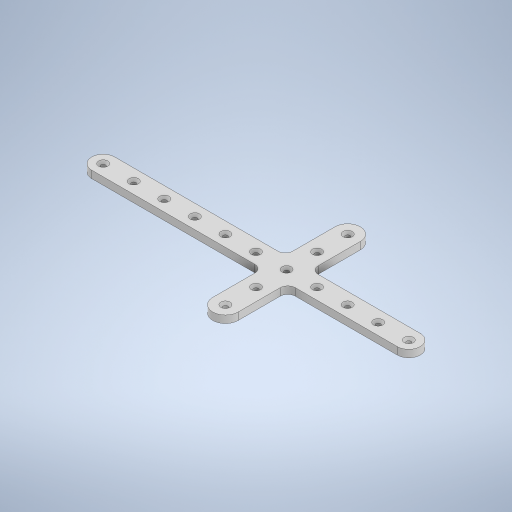
# Autodesk Inventor part: usztywnienie
Saved by Autodesk Inventor 2023.4 (Build 274418000, 418)
## iProperties
Created: 2024-07-31
Part Number: usztywnienie
Material: Generic
Document SubType Name: Modeling
Designer: komputer
Density: 1 g/cm^3
Appearance: Default
Author: komputer
Autodesk Inventor part; units mm, degrees
ref_plane "YZ Plane" through (0, 0, 0) normal (1, 0, 0) x (0, 1, 0)
ref_plane "XZ Plane" through (0, 0, 0) normal (0, 1, 0) x (-1, 0, 0)
ref_plane "XY Plane" through (0, 0, 0) normal (0, 0, 1) x (1, 0, 0)
sketch "Sketch1" plane through (0, 0, 0) normal (0, 1, 0) x (-1, 0, 0)
  circle A0 centre (-17.9853, 31.5522) radius 1.6
  circle A1 centre (22.0147, 11.5522) radius 1.6
  circle A2 centre (62.0147, 11.5522) radius 1.6
  circle A3 centre (102.0147, 11.5522) radius 1.6
  circle A4 centre (-17.9853, -8.4478) radius 1.6
  circle A5 centre (2.0147, 11.5522) radius 1.6
  circle A6 centre (-57.9853, 11.5522) radius 1.6
  circle A7 centre (-97.9853, 11.5522) radius 1.6
  circle A8 centre (-77.9853, 11.5522) radius 1.6
  circle A9 centre (-37.9853, 11.5522) radius 1.6
  circle A10 centre (-17.9853, -28.4478) radius 1.6
  circle A11 centre (-17.9853, 11.5522) radius 1.6
  circle A12 centre (-17.9853, 51.5522) radius 1.6
  circle A13 centre (82.0147, 11.5522) radius 1.6
  circle A14 centre (42.0147, 11.5522) radius 1.6
  line L0 (-9.6933, -37.4479) -> (-9.6933, -0.9478)
  arc A15 (-4.6933, 4.0522) -> (-9.6933, -0.9478) centre (-4.6933, -0.9478) ccw
  line L1 (-4.6933, 4.0522) -> (108.2535, 4.0522)
  line L2 (-26.2773, 59.9411) -> (-26.2773, 24.0522)
  arc A16 (-31.2773, 19.0522) -> (-26.2773, 24.0522) centre (-31.2773, 24.0522) ccw
  line L3 (-31.2773, 19.0522) -> (-110.8172, 19.0522)
  line L4 (-110.8172, 4.0522) -> (-31.2773, 4.0522)
  arc A17 (-26.2773, -0.9478) -> (-31.2773, 4.0522) centre (-31.2773, -0.9478) ccw
  line L5 (-26.2773, -0.9478) -> (-26.2773, -36.8367)
  line L6 (108.2535, 19.0522) -> (-4.6933, 19.0522)
  arc A18 (-9.6933, 24.0522) -> (-4.6933, 19.0522) centre (-4.6933, 24.0522) ccw
  line L7 (-9.6933, 24.0522) -> (-9.6933, 60.5523)
  circle A19 centre (-17.9853, 51.5522) radius 8.292
  circle A20 centre (-17.9853, -28.4478) radius 8.292
  circle A21 centre (102.0147, 11.5522) radius 7.5
  circle A22 centre (-97.9853, 11.5522) radius 7.5
  circle A23 centre (102.0147, 11.5522) radius 0.75
  circle A24 centre (82.0147, 11.5522) radius 0.75
  circle A25 centre (62.0147, 11.5522) radius 0.75
  circle A26 centre (42.0147, 11.5522) radius 0.75
  circle A27 centre (22.0147, 11.5522) radius 0.75
  circle A28 centre (2.0147, 11.5522) radius 0.75
  circle A29 centre (-17.9853, 11.5522) radius 0.75
  circle A30 centre (-37.9853, 11.5522) radius 0.75
  circle A31 centre (-57.9853, 11.5522) radius 0.75
  circle A32 centre (-77.9853, 11.5522) radius 0.75
  circle A33 centre (-97.9853, 11.5522) radius 0.75
  circle A34 centre (-17.9853, 51.5522) radius 0.75
  circle A35 centre (-17.9853, 31.5522) radius 0.75
  circle A36 centre (-17.9853, -8.4478) radius 0.75
  circle A37 centre (-17.9853, -28.4478) radius 0.75
  point P0 (0, 0)
  point P1 (-0.7536, 11.5522)
  point P2 (102.0147, 4.0522)
  point P3 (102.0147, 19.0522)
  point P4 (-9.6933, 51.5522)
  point P5 (-26.2773, 51.5522)
  point P6 (-97.9853, 19.0522)
  point P7 (-97.9853, 4.0522)
  point P8 (-26.2773, -28.4478)
  point P9 (-9.6933, -28.4478)
  dimension "d0" = 1.5
  dimension "d3" = 20
  dimension "d8" = 1.5
  dimension "d9" = 1.5
  dimension "d10" = 1.5
  dimension "d11" = 1.5
  constraints: 38 centre point, 16 end point, 9 coincident, 8 point on circle, 4 tangent, 1 horizontal, 20 other
  measures "d0" diameter of A23
  measures "d3" distance of A23.centre A24.centre
  measures "d8" diameter of A34
  measures "d9" diameter of A35
  measures "d10" diameter of A36
  measures "d11" diameter of A37
extrude "Extrusion1" add sketch "Sketch1" along normal blind 4.8 contours A0 | A1 | A2 | A3 | A4 | A5 | A6 | A7 | A8 | A9 | A10 | A11 | A12 | A13 | A14 | A20 L5 A17 L4 A22 L3 A16 L2 A19 L7 A18 L6 A21 L1 A15 L0 | A20 | A21 | A22 | A19
sketch "Sketch3" plane through (0, 4.8, 0) normal (0, 1, 0) x (1, 0, 0)
  line L0 (-102.0147, -19.0522) -> (4.6933, -19.0522) projected
  arc A0 (9.6933, -24.0522) -> (4.6933, -19.0522) centre (4.6933, -24.0522) ccw projected
  line L1 (9.6933, -24.0522) -> (9.6933, -51.5522) projected
  arc A1 (9.6933, -51.5522) -> (26.2773, -51.5522) centre (17.9853, -51.5522) ccw projected
  line L2 (26.2773, -51.5522) -> (26.2773, -24.0522) projected
  arc A2 (31.2773, -19.0522) -> (26.2773, -24.0522) centre (31.2773, -24.0522) ccw projected
  line L3 (31.2773, -19.0522) -> (97.9853, -19.0522) projected
  arc A3 (97.9853, -19.0522) -> (97.9853, -4.0522) centre (97.9853, -11.5522) ccw projected
  line L4 (97.9853, -4.0522) -> (31.2773, -4.0522) projected
  arc A4 (26.2773, 0.9478) -> (31.2773, -4.0522) centre (31.2773, 0.9478) ccw projected
  line L5 (26.2773, 0.9478) -> (26.2773, 28.4478) projected
  arc A5 (26.2773, 28.4478) -> (9.6933, 28.4478) centre (17.9853, 28.4478) ccw projected
  line L6 (9.6933, 28.4478) -> (9.6933, 0.9478) projected
  arc A6 (4.6933, -4.0522) -> (9.6933, 0.9478) centre (4.6933, 0.9478) ccw projected
  line L7 (4.6933, -4.0522) -> (-102.0147, -4.0522) projected
  arc A7 (-102.0147, -4.0522) -> (-102.0147, -19.0522) centre (-102.0147, -11.5522) ccw projected
  circle A8 centre (17.9853, 28.4478) radius 0.75 projected
  circle A9 centre (97.9853, -11.5522) radius 0.75 projected
  circle A10 centre (17.9853, -51.5522) radius 0.75 projected
  circle A11 centre (17.9853, -31.5522) radius 0.75 projected
  circle A12 centre (17.9853, -11.5522) radius 0.75 projected
  circle A13 centre (17.9853, 8.4478) radius 0.75 projected
  circle A14 centre (37.9853, -11.5522) radius 0.75 projected
  circle A15 centre (77.9853, -11.5522) radius 0.75 projected
  circle A16 centre (57.9853, -11.5522) radius 0.75 projected
  circle A17 centre (-42.0147, -11.5522) radius 0.75 projected
  circle A18 centre (-2.0147, -11.5522) radius 0.75 projected
  circle A19 centre (-22.0147, -11.5522) radius 0.75 projected
  circle A20 centre (-82.0147, -11.5522) radius 0.75 projected
  circle A21 centre (-62.0147, -11.5522) radius 0.75 projected
  circle A22 centre (-102.0147, -11.5522) radius 0.75 projected
  point P0 (0, 0)
hole "Hole1" at (-102.0147, 4.8, 11.5522) at (-82.0147, 4.8, 11.5522) at (-62.0147, 4.8, 11.5522) at (-42.0147, 4.8, 11.5522) at (-22.0147, 4.8, 11.5522) at (-2.0147, 4.8, 11.5522) at (17.9853, 4.8, -28.4478) at (17.9853, 4.8, -8.4478) at (17.9853, 4.8, 11.5522) at (17.9853, 4.8, 31.5522) at (37.9853, 4.8, 11.5522) at (17.9853, 4.8, 51.5522) at (57.9853, 4.8, 11.5522) at (77.9853, 4.8, 11.5522) at (97.9853, 4.8, 11.5522) direction (0, -1, 0) diameter 3 end through all countersink diameter 6 countersink angle 90
body "Solid1"
